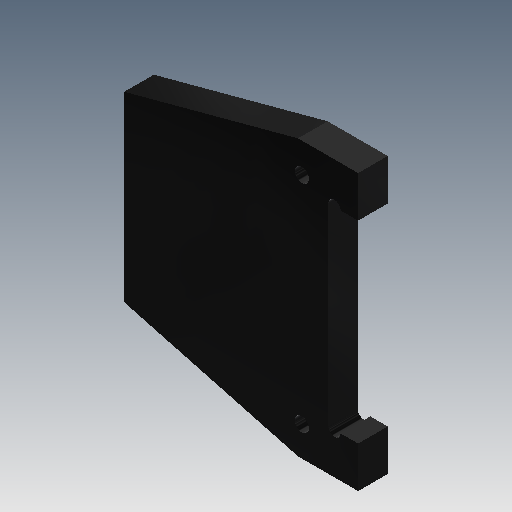
# Autodesk Inventor part: 胴体_サブフレーム_1_7
Saved by Autodesk Inventor 2017.3 (Build 213256000, 256)
## iProperties
Created: 2016-05-15
Part Number: 胴体_サブフレーム_1_7
Material: アセタール樹脂、黒
Document SubType Name: Modeling
Designer: hiroaki
Density: 1.425 g/cm^3
Appearance: 滑らか - 黒
Mass: 6.61533 g
Surface Area: 42.3195 cm^2
Volume: 4.64234 cm^3
Author: hiroaki
Autodesk Inventor part; units mm, degrees
ref_plane "YZ Plane" through (0, 0, 0) normal (1, 0, 0) x (0, 1, 0)
ref_plane "XZ Plane" through (0, 0, 0) normal (0, 1, 0) x (-1, 0, 0)
ref_plane "XY Plane" through (0, 0, 0) normal (0, 0, 1) x (1, 0, 0)
sketch "スケッチ1" plane through (0, 0, 0) normal (0, 0, 1) x (1, 0, 0)
  line L0 (0, 16.25) -> (28.465632, 16.25) construction
  line L1 (28.465632, 16.25) -> (28.465632, -16.25) construction
  line L2 (28.465632, -16.25) -> (0, -16.25) construction
  line L3 (0, -16.25) -> (0, 16.25) construction
  line L4 (5, 23.25) -> (-5.158262, 23.25)
  line L5 (-5.158262, 23.25) -> (-34.5, 15.387905)
  line L6 (-34.5, 15.387905) -> (-34.5, -15.387905)
  line L7 (-34.5, -15.387905) -> (-5.158262, -23.25)
  line L8 (-5.158262, -23.25) -> (5, -23.25)
  line L9 (5, -23.25) -> (5, -16.3)
  line L10 (5, -16.3) -> (2.05, -16.3)
  arc A0 (-0.05, -16.3) -> (2.05, -16.3) centre (1, -16.3) ccw
  line L11 (-0.05, -16.3) -> (-0.05, 16.3)
  arc A1 (2.05, 16.3) -> (-0.05, 16.3) centre (1, 16.3) ccw
  line L12 (28.465632, 0) -> (0, 0) construction
  line L13 (2.05, 16.3) -> (5, 16.3)
  line L14 (5, 16.3) -> (5, 23.25)
  line L15 (28.515632, 16.3) -> (-0.05, 16.3) construction
  line L16 (-0.05, 16.3) -> (-0.05, -16.3) construction
  line L17 (-0.05, -16.3) -> (28.515632, -16.3) construction
  line L18 (28.515632, -16.3) -> (28.515632, 16.3) construction
  circle A2 centre (-4.5, 18.25) radius 1.2
  circle A3 centre (-4.5, -18.25) radius 1.2
  line L19 (0, 0) -> (28.465632, 0) construction
  line L20 (2.5, 16.25) -> (2.5, -16.25) construction
  circle A4 centre (-4.5, 18.25) radius 5 construction
  line L21 (-6.087713, 15.5) -> (-7.675426, 18.25)
  line L22 (-7.675426, 18.25) -> (-6.087713, 21)
  line L23 (-6.087713, 21) -> (-2.912287, 21)
  line L24 (-2.912287, 21) -> (-1.324574, 18.25)
  line L25 (-1.324574, 18.25) -> (-2.912287, 15.5)
  line L26 (-2.912287, 15.5) -> (-6.087713, 15.5)
  point P0 (-34.5, 0)
  point P1 (-0.05, 0)
  dimension "d98" = 32.5
  dimension "d100" = 0.05
  dimension "d101" = 1.05
  dimension "d102" = 5
  dimension "d104" = 2.4
  dimension "d106" = 2.5
  dimension "d107" = 7
  dimension "d108" = 18.25
  dimension "d109" = 5
  dimension "d110" = 30
  dimension "d111" = 165
  dimension "d130" = 5.5
  constraints: 54 end point, 6 equal length, 5 centre point, 4 coincident, 4 horizontal, 4 midpoint, 4 perpendicular, 4 point on circle, 4 point on line, 4 tangent, 3 collinear, 3 symmetric about line, 3 vertical, 2 equal radius, 1 horizontal alignment, 1 vertical alignment, 17 other
  measures "d98" distance of L0.end L1.end
  measures "d100" distance between parallel lines of L0 L15
  measures "d101" radius of A0
  measures "d102" distance between parallel lines of L14 L3
  measures "d104" diameter of A2
  measures "d106" distance between parallel lines of L20 L3
  measures "d107" distance from line of A2.centre L20
  measures "d108" distance from line of L12 A2.centre
  measures "d109" distance from line of A2.centre L4
  measures "d110" distance from line of A2.centre L6
  measures "d111" angle of L4 L5
  measures "d130" distance between parallel lines of L26 L23
extrude "押し出し1" add sketch "スケッチ1" along normal blind 5 contours L14 L13 A1 L11 A0 L10 L9 L8 L7 L6 L5 L4 | L21 L22 L23 L24 L25 L26
sketch "スケッチ6" plane through (0, 0, 0) normal (0, 0, -1) x (-1, 0, 0)
  line L0 (34.5, -15.387905) -> (5.158262, -23.25)
  line L1 (34.5, 15.387905) -> (34.5, -15.387905)
  line L2 (5.158262, 23.25) -> (34.5, 15.387905)
  line L3 (8.5, 17.178203) -> (8.5, -17.178203)
  line L4 (8.5, -17.178203) -> (29.5, -11.55127)
  line L5 (29.5, -11.55127) -> (29.5, 11.55127)
  line L6 (29.5, 11.55127) -> (8.5, 17.178203)
  circle A0 centre (4.5, 18.25) radius 1.2
  point P0 (0, 0)
  dimension "d113" = 5
  dimension "d114" = 5
  dimension "d115" = 5
  dimension "d133" = 4
  constraints: 8 end point, 3 parallel, 1 vertical
  measures "d113" distance between parallel lines of L2 L6
  measures "d114" distance between parallel lines of L0 L4
  measures "d115" distance between parallel lines of L1 L5
  measures "d133" distance from line of A0.centre L3
extrude "押し出し4" cut sketch "スケッチ6" against normal blind 4 contours L6 L5 L4 L3
fillet "フィレット2" radius 1.05 4 edges at (-8.5, 17.1782, 2) (-8.5, -17.1782, 2) (-29.5, 11.5513, 2) (-29.5, -11.5513, 2)
sketch "スケッチ7" plane through (0, 0, 0) normal (0, 0, -1) x (-1, 0, 0)
  circle A0 centre (4.5, -18.25) radius 1.2
  circle A1 centre (4.5, 18.25) radius 1.2
  line L0 (2.912287, 15.5) -> (1.324574, 18.25)
  line L1 (1.324574, 18.25) -> (2.912287, 21)
  line L2 (2.912287, 21) -> (6.087713, 21)
  line L3 (6.087713, 21) -> (7.675426, 18.25)
  line L4 (7.675426, 18.25) -> (6.087713, 15.5)
  line L5 (6.087713, 15.5) -> (2.912287, 15.5)
  line L6 (7.6812, 18.25) -> (6.0906, 21.005)
  line L7 (6.0906, 21.005) -> (2.9094, 21.005)
  line L8 (2.9094, 21.005) -> (1.3188, 18.25)
  line L9 (1.3188, 18.25) -> (2.9094, 15.495)
  line L10 (2.9094, 15.495) -> (6.0906, 15.495)
  line L11 (6.0906, 15.495) -> (7.6812, 18.25)
  circle A2 centre (6.6312, 18.25) radius 1.05
  circle A3 centre (5.5656, 20.095673) radius 1.05
  circle A4 centre (3.4344, 20.095673) radius 1.05
  circle A5 centre (2.3688, 18.25) radius 1.05
  circle A6 centre (3.4344, 16.404327) radius 1.05
  circle A7 centre (5.5656, 16.404327) radius 1.05
  line L12 (7.6812, -18.25) -> (6.0906, -21.005)
  line L13 (6.0906, -21.005) -> (2.9094, -21.005)
  line L14 (2.9094, -21.005) -> (1.3188, -18.25)
  line L15 (1.3188, -18.25) -> (2.9094, -15.495)
  line L16 (2.9094, -15.495) -> (6.0906, -15.495)
  line L17 (6.0906, -15.495) -> (7.6812, -18.25)
  circle A8 centre (6.6312, -18.25) radius 1.05
  circle A9 centre (5.5656, -16.404327) radius 1.05
  circle A10 centre (3.4344, -16.404327) radius 1.05
  circle A11 centre (2.3688, -18.25) radius 1.05
  circle A12 centre (3.4344, -20.095673) radius 1.05
  circle A13 centre (5.5656, -20.095673) radius 1.05
  point P0 (0, 0)
  point P1 (6.0906, 21.005)
  point P2 (2.9094, 21.005)
  point P3 (1.3188, 18.25)
  point P4 (2.9094, 15.495)
  point P5 (6.0906, 15.495)
  point P6 (2.9094, -15.495)
  point P7 (2.9094, -21.005)
  point P8 (6.0906, -21.005)
  dimension "d121" = 2.1
  dimension "d119" = 5.5
  dimension "d120" = 0.005
  dimension "d124" = 360
  dimension "d128" = 360
  constraints: 36 end point, 6 horizontal alignment, 2 coincident, 2 horizontal, 1 parallel, 101 other
  measures "d119" distance between parallel lines of L5 L2
  measures "d120" distance between parallel lines of L6 L3
sketch "スケッチ7 outline for 押し出し5" plane through (0, 0, 0) normal (0, 0, -1) x (-1, 0, 0)
  arc A0 (6.6156, 20.095673) -> (5.0406, 21.005) centre (5.5656, 20.095673) ccw
  line L0 (5.0406, 21.005) -> (3.9594, 21.005)
  arc A1 (3.9594, 21.005) -> (2.3844, 20.095673) centre (3.4344, 20.095673) ccw
  line L1 (2.3844, 20.095673) -> (1.8438, 19.159327)
  arc A2 (1.8438, 19.159327) -> (1.8438, 17.340673) centre (2.3688, 18.25) ccw
  line L2 (1.8438, 17.340673) -> (2.3844, 16.404327)
  arc A3 (2.3844, 16.404327) -> (3.9594, 15.495) centre (3.4344, 16.404327) ccw
  line L3 (3.9594, 15.495) -> (5.0406, 15.495)
  arc A4 (5.0406, 15.495) -> (6.6156, 16.404327) centre (5.5656, 16.404327) ccw
  line L4 (6.6156, 16.404327) -> (7.1562, 17.340673)
  arc A5 (7.1562, 17.340673) -> (7.1562, 19.159327) centre (6.6312, 18.25) ccw
  line L5 (7.1562, 19.159327) -> (6.6156, 20.095673)
  arc A6 (6.6156, -16.404327) -> (5.0406, -15.495) centre (5.5656, -16.404327) ccw
  line L6 (3.9594, -15.495) -> (5.0406, -15.495)
  arc A7 (3.9594, -15.495) -> (2.3844, -16.404327) centre (3.4344, -16.404327) ccw
  line L7 (1.8438, -17.340673) -> (2.3844, -16.404327)
  arc A8 (1.8438, -17.340673) -> (1.8438, -19.159327) centre (2.3688, -18.25) ccw
  line L8 (2.3844, -20.095673) -> (1.8438, -19.159327)
  arc A9 (2.3844, -20.095673) -> (3.9594, -21.005) centre (3.4344, -20.095673) ccw
  line L9 (5.0406, -21.005) -> (3.9594, -21.005)
  arc A10 (5.0406, -21.005) -> (6.6156, -20.095673) centre (5.5656, -20.095673) ccw
  line L10 (7.1562, -19.159327) -> (6.6156, -20.095673)
  arc A11 (7.1562, -19.159327) -> (7.1562, -17.340673) centre (6.6312, -18.25) ccw
  line L11 (6.6156, -16.404327) -> (7.1562, -17.340673)
  arc A12 (5.644781, -17.890171) -> (5.384012, -17.438505) centre (4.5, -18.25) ccw
  arc A13 (5.644781, -17.890171) -> (5.644781, -18.609829) centre (6.6312, -18.25) ccw
  arc A14 (5.384012, -19.061495) -> (5.644781, -18.609829) centre (4.5, -18.25) ccw
  arc A15 (5.384012, -19.061495) -> (4.760769, -19.421324) centre (5.5656, -20.095673) ccw
  arc A16 (4.239231, -19.421324) -> (4.760769, -19.421324) centre (4.5, -18.25) ccw
  arc A17 (4.239231, -19.421324) -> (3.615988, -19.061495) centre (3.4344, -20.095673) ccw
  arc A18 (3.355219, -18.609829) -> (3.615988, -19.061495) centre (4.5, -18.25) ccw
  arc A19 (3.355219, -18.609829) -> (3.355219, -17.890171) centre (2.3688, -18.25) ccw
  arc A20 (3.615988, -17.438505) -> (3.355219, -17.890171) centre (4.5, -18.25) ccw
  arc A21 (3.615988, -17.438505) -> (4.239231, -17.078676) centre (3.4344, -16.404327) ccw
  arc A22 (4.760769, -17.078676) -> (4.239231, -17.078676) centre (4.5, -18.25) ccw
  arc A23 (4.760769, -17.078676) -> (5.384012, -17.438505) centre (5.5656, -16.404327) ccw
extrude "押し出し5" cut sketch "スケッチ7 outline for 押し出し5" against normal blind 2
equation "\"d114\" = d113"
equation "\"d115\" = d113"
